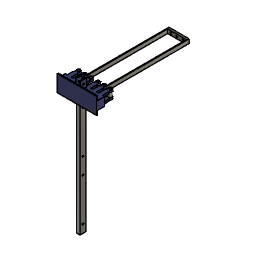
Modelo Dinamica De Estructuras (Autodesk Fusion 360 design; units mm, degrees)
Autodesk Fusion 360 part; units mm, degrees
note: some values were not read from the file. Set by a fixed rule: which sketch regions a step uses.
sketch "Boceto1" plane through (0, 0, 0) normal (0, 0, 1) x (1, 0, 0)
  circle A0 centre (0, 0) radius 2.65
  circle A1 centre (48, 0) radius 2.65
  circle A2 centre (0, 0) radius 5
  circle A3 centre (48, 0) radius 5
  line L0 (-25, -8) -> (73, -8)
  line L1 (73, -8) -> (73, -18)
  line L2 (73, -18) -> (-25, -18)
  line L3 (-25, -18) -> (-25, -8)
  line L4 (0, 0) -> (-5, -8)
  line L5 (0, 0) -> (5, -8)
  line L6 (48, 0) -> (43, -8)
  line L7 (48, 0) -> (53, -8)
  line L8 (0, 0) -> (48, 0) construction
  circle A4 centre (15, 0) radius 2.65
  circle A5 centre (15, 0) radius 5
  circle A6 centre (33, 0) radius 2.65
  circle A7 centre (33, 0) radius 5
  circle A8 centre (63, 0) radius 2.65
  circle A9 centre (63, 0) radius 5
  circle A10 centre (-15, 0) radius 5
  circle A11 centre (-15, 0) radius 2.65
  line L9 (-15, 5) -> (63, 5) construction
  line L10 (-15, 2.65) -> (63, 2.65) construction
  line L11 (-15, 0) -> (0, 0) construction
  line L12 (63, 0) -> (48, 0) construction
  line L13 (-15, 0) -> (-20, -8)
  line L14 (-15, 0) -> (-10, -8)
  line L15 (15, 0) -> (10, -8)
  line L16 (15, 0) -> (20, -8)
  line L17 (33, 0) -> (28, -8)
  line L18 (33, 0) -> (38, -8)
  line L19 (63, 0) -> (58, -8)
  line L20 (63, 0) -> (68, -8)
  dimension "d1" = 5.3
  dimension "d6" = 10
  dimension "d8" = 8
  dimension "d11" = 48
  dimension "d16" = 15
  dimension "d17" = 15
  dimension "d18" = 15
  dimension "d19" = 15
  dimension "d20" = 98
  dimension "d21" = 10
  dimension "d22" = 25
  constraint coincident A0.centre A2.centre
  constraint concentric A0 A2
  constraint concentric A1 A3
  constraint horizontal L0
  constraint vertical L1
  constraint horizontal L2
  constraint vertical L3
  constraint coincident L0 L4.end
  constraint coincident L0 L5.end
  constraint coincident A1.centre A3.centre
  constraint coincident L0 L6.end
  constraint coincident L0 L7.end
  constraint parallel L5 L7
  constraint equal L4 L5
  constraint equal L6 L7
  constraint horizontal L8
  constraint coincident L8 A4.centre
  constraint concentric A4 A5
  constraint coincident L8 A6.centre
  constraint concentric A6 A7
  constraint concentric A8 A9
  constraint concentric A10 A11
  constraint coincident A10 L9.start
  constraint horizontal L9
  constraint coincident A11 L10.start
  constraint horizontal L10
  constraint tangent A0 L10
  constraint tangent A2 L9
  constraint tangent A5 L9
  constraint tangent A4 L10
  constraint tangent A6 L10
  constraint tangent A7 L9
  constraint tangent A3 L9
  constraint tangent A1 L10
  constraint tangent A8 L10
  constraint tangent A9 L9
  constraint tangent A10 L9
  constraint tangent A11 L10
  constraint coincident A10.centre A11.centre
  constraint coincident A8.centre A9.centre
  constraint horizontal L12
  constraint horizontal L11
  constraint coincident A8 L10.end
  constraint coincident A9 L9.end
  constraint coincident L0 L13.end
  constraint coincident L0 L14.end
  constraint coincident A4.centre A5.centre
  constraint coincident L0 L15.end
  constraint coincident L0 L16.end
  constraint parallel L14 L16
  constraint coincident A6.centre A7.centre
  constraint coincident L0 L17.end
  constraint parallel L15 L17
  constraint coincident L0 L18.end
  constraint parallel L16 L18
  constraint coincident L0 L19.end
  constraint parallel L17 L19
  constraint coincident L0 L20.end
  constraint parallel L18 L20
  constraint equal L13 L14
  constraint equal L4 L14
  constraint equal L15 L16
  measures "d1" diameter of A0
  measures "d6" diameter of A2
  measures "d8" distance of A0.centre L0
  measures "d11" distance of A1.centre A0.centre
  measures "d16" distance of A0.centre A10.centre
  measures "d17" distance of A0.centre A4.centre
  measures "d18" distance of A1.centre A6.centre
  measures "d19" distance of A1.centre A8.centre
  measures "d20" distance of L1.end L2.end
  measures "d21" distance of L0.start L2.end
  measures "d22" distance of A0.centre L3
extrude "Extruir1" add sketch "Boceto1" along normal blind 21 contours A0 A2 L4 L5 | A0 A2 L4 L5 | A2 L0 L4 L5 | L0 L1 L2 L3 | L0 A10 L13 L14 | L0 A5 L15 L16 | A10 A11 L13 L14 | A10 A11 L13 L14 | A4 A5 L15 L16 | A4 A5 L15 L16 | L0 A7 L17 L18 | A6 A7 L17 L18 | A6 A7 L17 L18 | A3 L0 L6 L7 | A1 A3 L6 L7 | A1 A3 L6 L7 | L0 A9 L19 L20 | A8 A9 L19 L20 | A8 A9 L19 L20 makes body 1
sketch "Boceto2" plane through (-25, 0, 0) normal (-1, 0, 0) x (0, -1, 0)
  line L0 (8, 0) -> (18, 0)
  line L1 (18, 0) -> (18, 21)
  line L2 (18, 21) -> (8, 21)
  line L3 (8, 21) -> (8, 0)
  line L4 (8, 10.5) -> (-7.6781, 10.5)
  line L5 (-7.6781, 10.5) -> (-7.6781, 5)
  line L6 (-7.6781, 5) -> (8, 5)
  line L7 (8, 5) -> (8, 10.5)
  line L8 (8, 10.5) -> (-7.9551, 10.5)
  line L9 (-7.9551, 10.5) -> (-7.9551, 16)
  line L10 (-7.9551, 16) -> (8, 16)
  line L11 (8, 16) -> (8, 10.5)
  dimension "d23" = 11
  constraint horizontal L4
  constraint vertical L5
  constraint horizontal L6
  constraint vertical L7
  constraint midpoint L3 L4.start
  constraint horizontal L8
  constraint vertical L9
  constraint horizontal L10
  constraint vertical L11
  constraint equal L7 L11
  measures "d23" distance of L6 L10
extrude "Extruir2" cut sketch "Boceto2" against normal through all contours L3 L4 L5 L6 L7 L8 | L3 L4 L8 L9 L10 L11 bodies 1
extrude "Extruir3" add sketch "Boceto1" along normal blind 1 contours A3 L0 L6 L7 bodies 1
sketch "Boceto4" plane through (0, 0, 0) normal (0, 0, -1) x (1, 0, 0)
  circle A0 centre (48, 0) radius 3
  circle A1 centre (0, 0) radius 3
  circle A2 centre (63, 0) radius 3
  circle A3 centre (15, 0) radius 3
  circle A4 centre (33, 0) radius 3
  arc A5 (-17.65, 4.24) -> (-12.35, 4.24) centre (-15, 0) ccw
  line L0 (-12.35, 4.24) -> (-10, 8)
  line L1 (-10, 8) -> (-5, 8)
  line L2 (-5, 8) -> (-2.65, 4.24)
  arc A6 (-2.65, 4.24) -> (2.65, 4.24) centre (0, 0) ccw
  line L3 (2.65, 4.24) -> (5, 8)
  line L4 (5, 8) -> (10, 8)
  line L5 (10, 8) -> (12.35, 4.24)
  arc A7 (12.35, 4.24) -> (17.65, 4.24) centre (15, 0) ccw
  line L6 (17.65, 4.24) -> (20, 8)
  line L7 (20, 8) -> (28, 8)
  line L8 (28, 8) -> (30.35, 4.24)
  arc A8 (30.35, 4.24) -> (35.65, 4.24) centre (33, 0) ccw
  line L9 (35.65, 4.24) -> (38, 8)
  line L10 (38, 8) -> (43, 8)
  line L11 (43, 8) -> (45.35, 4.24)
  arc A9 (45.35, 4.24) -> (50.65, 4.24) centre (48, 0) ccw
  line L12 (50.65, 4.24) -> (53, 8)
  line L13 (53, 8) -> (58, 8)
  line L14 (58, 8) -> (60.35, 4.24)
  arc A10 (60.35, 4.24) -> (65.65, 4.24) centre (63, 0) ccw
  line L15 (65.65, 4.24) -> (68, 8)
  line L16 (68, 8) -> (73, 8)
  line L17 (73, 8) -> (73, 18)
  line L18 (73, 18) -> (-25, 18)
  line L19 (-25, 18) -> (-25, 8)
  line L20 (-25, 8) -> (-20, 8)
  line L21 (-20, 8) -> (-17.65, 4.24)
  circle A11 centre (-15, 0) radius 3
  circle A12 centre (48, 13) radius 4
  circle A13 centre (0, 13) radius 4
  line L22 (48, 0) -> (48, 13) construction
  line L23 (0, 0) -> (0, 13) construction
  line L24 (48, 13) -> (0, 13) construction
  dimension "d36" = 5.2
  dimension "d37" = 8
  dimension "d38" = 8
  constraint coincident A0.centre A9.centre
  constraint coincident A12.centre L22.end
  constraint coincident A1.centre A6.centre
  constraint coincident A13.centre L23.end
  constraint vertical L23
  constraint vertical L22
  constraint horizontal L24
  measures "d37" diameter of A12
  measures "d38" diameter of A13
extrude "Extruir5" [suppressed]
sketch "Boceto5" plane through (0, 0, 0) normal (0, 0, -1) x (1, 0, 0)
  circle A0 centre (48, 0) radius 2.65
  circle A1 centre (0, 0) radius 2.65
  circle A2 centre (63, 0) radius 2.65
  circle A3 centre (15, 0) radius 2.65
  circle A4 centre (33, 0) radius 2.65
  arc A5 (-17.65, 4.24) -> (-12.35, 4.24) centre (-15, 0) ccw
  line L0 (-12.35, 4.24) -> (-10, 8)
  line L1 (-10, 8) -> (-5, 8)
  line L2 (-5, 8) -> (-2.65, 4.24)
  arc A6 (-2.65, 4.24) -> (2.65, 4.24) centre (0, 0) ccw
  line L3 (2.65, 4.24) -> (5, 8)
  line L4 (5, 8) -> (10, 8)
  line L5 (10, 8) -> (12.35, 4.24)
  arc A7 (12.35, 4.24) -> (17.65, 4.24) centre (15, 0) ccw
  line L6 (17.65, 4.24) -> (20, 8)
  line L7 (20, 8) -> (28, 8)
  line L8 (28, 8) -> (30.35, 4.24)
  arc A8 (30.35, 4.24) -> (35.65, 4.24) centre (33, 0) ccw
  line L9 (35.65, 4.24) -> (38, 8)
  line L10 (38, 8) -> (43, 8)
  line L11 (43, 8) -> (45.35, 4.24)
  arc A9 (45.35, 4.24) -> (50.65, 4.24) centre (48, 0) ccw
  line L12 (50.65, 4.24) -> (53, 8)
  line L13 (53, 8) -> (58, 8)
  line L14 (58, 8) -> (60.35, 4.24)
  arc A10 (60.35, 4.24) -> (65.65, 4.24) centre (63, 0) ccw
  line L15 (65.65, 4.24) -> (68, 8)
  line L16 (68, 8) -> (73, 8)
  line L17 (73, 8) -> (73, 18)
  line L18 (73, 18) -> (-25, 18)
  line L19 (-25, 18) -> (-25, 8)
  line L20 (-25, 8) -> (-20, 8)
  line L21 (-20, 8) -> (-17.65, 4.24)
  circle A11 centre (-15, 0) radius 2.65
  line L22 (73, 18) -> (-25, 18)
  line L23 (-25, 18) -> (-25, 8)
  line L24 (-25, 8) -> (73, 8)
  line L25 (73, 8) -> (73, 18)
  constraint horizontal L22
  constraint vertical L23
  constraint horizontal L24
  constraint vertical L25
  constraint coincident L19.end L20.start
  constraint coincident L17.end L18.start
extrude "Extruir6" add sketch "Boceto5" along normal blind 50 separate body contours L1 L4 L7 L10 L13 L16 L17 L18 L19 L20 L22 L23 L24 L25 makes body 2
pattern_linear "Patrón R2" count 3 spacing 80 along (0, 0, -1) of bodies 1 makes body 3 at (40.3333, -18, -73) makes body 4 at (40.3333, -18, -153)
pattern_linear "Patrón R3" count 2 spacing 80 along (0, 0, -1) of bodies 2 makes body 5
sketch "Boceto6" plane through (0, 0, -160) normal (0, 0, -1) x (1, 0, 0)
  circle A0 centre (48, 13) radius 4
  circle A1 centre (0, 13) radius 4
  circle A2 centre (48, 0) radius 3
  circle A3 centre (0, 0) radius 3
  circle A4 centre (63, 0) radius 3
  circle A5 centre (15, 0) radius 3
  circle A6 centre (33, 0) radius 3
  arc A7 (-17.65, 4.24) -> (-12.35, 4.24) centre (-15, 0) ccw
  line L0 (-12.35, 4.24) -> (-10, 8)
  line L1 (-10, 8) -> (-5, 8)
  line L2 (-5, 8) -> (-2.65, 4.24)
  arc A8 (-2.65, 4.24) -> (2.65, 4.24) centre (0, 0) ccw
  line L3 (2.65, 4.24) -> (5, 8)
  line L4 (5, 8) -> (10, 8)
  line L5 (10, 8) -> (12.35, 4.24)
  arc A9 (12.35, 4.24) -> (17.65, 4.24) centre (15, 0) ccw
  line L6 (17.65, 4.24) -> (20, 8)
  line L7 (20, 8) -> (28, 8)
  line L8 (28, 8) -> (30.35, 4.24)
  arc A10 (30.35, 4.24) -> (35.65, 4.24) centre (33, 0) ccw
  line L9 (35.65, 4.24) -> (38, 8)
  line L10 (38, 8) -> (43, 8)
  line L11 (43, 8) -> (45.35, 4.24)
  arc A11 (45.35, 4.24) -> (50.65, 4.24) centre (48, 0) ccw
  line L12 (50.65, 4.24) -> (53, 8)
  line L13 (53, 8) -> (58, 8)
  line L14 (58, 8) -> (60.35, 4.24)
  arc A12 (60.35, 4.24) -> (65.65, 4.24) centre (63, 0) ccw
  line L15 (65.65, 4.24) -> (68, 8)
  line L16 (68, 8) -> (73, 8)
  line L17 (73, 8) -> (73, 18)
  line L18 (73, 18) -> (-25, 18)
  line L19 (-25, 18) -> (-25, 8)
  line L20 (-25, 8) -> (-20, 8)
  line L21 (-20, 8) -> (-17.65, 4.24)
  circle A13 centre (-15, 0) radius 3
  circle A14 centre (63, 0) radius 3
  circle A15 centre (48, 0) radius 3
  circle A16 centre (33, 0) radius 3
  circle A17 centre (15, 0) radius 3
  circle A18 centre (0, 0) radius 3
  circle A19 centre (-15, 0) radius 3
  circle A20 centre (0, 13) radius 4
  circle A21 centre (48, 13) radius 4
extrude "Extruir7" [suppressed]
sketch "Boceto7" plane through (0, 0, 16) normal (0, 0, -1) x (1, 0, 0)
  arc A0 (60.35, 4.24) -> (65.65, 4.24) centre (63, 0) ccw
  circle A1 centre (63, 0) radius 2.65
  circle A2 centre (48, 0) radius 2.65
  arc A3 (45.35, 4.24) -> (50.65, 4.24) centre (48, 0) ccw
  arc A4 (30.35, 4.24) -> (35.65, 4.24) centre (33, 0) ccw
  circle A5 centre (33, 0) radius 2.65
  arc A6 (12.35, 4.24) -> (17.65, 4.24) centre (15, 0) ccw
  circle A7 centre (15, 0) radius 2.65
  arc A8 (-2.65, 4.24) -> (2.65, 4.24) centre (0, 0) ccw
  circle A9 centre (0, 0) radius 2.65
  arc A10 (-17.65, 4.24) -> (-12.35, 4.24) centre (-15, 0) ccw
  circle A11 centre (-15, 0) radius 2.65
  arc A12 (60.456, 4.0704) -> (60.4559, 4.0703) centre (63, 0) ccw
  arc A13 (60.4559, 4.0703) -> (60.456, 4.0704) centre (57.912, 8.1408) ccw
  circle A14 centre (48, 0) radius 4.8
  circle A15 centre (33, 0) radius 4.8
  circle A16 centre (15, 0) radius 4.8
  circle A17 centre (0, 0) radius 4.8
  circle A18 centre (-15, 0) radius 4.8
  line L0 (63, 0) -> (-15, 0) construction
  line L1 (58.4404, -1.5) -> (52.5596, -1.5)
  line L2 (58.4404, 1.5) -> (52.5596, 1.5)
  line L3 (43.4404, -1.5) -> (37.5596, -1.5)
  line L4 (43.4404, 1.5) -> (37.5596, 1.5)
  line L5 (10.4404, -1.5) -> (4.5596, -1.5)
  line L6 (10.4404, 1.5) -> (4.5596, 1.5)
  line L7 (-4.5596, -1.5) -> (-10.4404, -1.5)
  line L8 (-4.5596, 1.5) -> (-10.4404, 1.5)
  line L9 (48, -4.8) -> (0, -4.8) construction
  line L10 (0, -4.8) -> (0, -204.8) construction
  line L11 (0, -204.8) -> (48, -204.8)
  line L12 (48, -204.8) -> (48, -4.8) construction
  line L13 (47, -204.8) -> (47, -4.6947)
  line L14 (49, -204.8) -> (49, -4.6947)
  line L15 (1, -204.8) -> (1, -4.6947)
  line L16 (-1, -204.8) -> (-1, -4.6947)
  line L17 (49, -204.8) -> (-1, -204.8)
  line L18 (-1, -204.8) -> (-1, -210)
  line L19 (-1, -210) -> (49, -210)
  line L20 (49, -210) -> (49, -204.8)
  line L21 (65.65, 4.24) -> (68, 8)
  line L22 (68, 8) -> (58, 8)
  line L23 (58, 8) -> (60.35, 4.24)
  line L24 (35.65, 4.24) -> (38, 8)
  line L25 (38, 8) -> (28, 8)
  line L26 (28, 8) -> (30.35, 4.24)
  line L27 (17.65, 4.24) -> (20, 8)
  line L28 (20, 8) -> (10, 8)
  line L29 (10, 8) -> (12.35, 4.24)
  line L30 (-12.35, 4.24) -> (-10, 8)
  line L31 (-10, 8) -> (-20, 8)
  line L32 (-20, 8) -> (-17.65, 4.24)
  line L33 (50.65, 4.24) -> (53, 8)
  line L34 (53, 8) -> (43, 8)
  line L35 (43, 8) -> (45.35, 4.24)
  line L36 (2.65, 4.24) -> (5, 8)
  line L37 (5, 8) -> (-5, 8)
  line L38 (-5, 8) -> (-2.65, 4.24)
  circle A19 centre (63, 0) radius 4.8
  dimension "d56" = 3
  dimension "d58" = 200
  dimension "d59" = 2
  dimension "d60" = 1
  dimension "d61" = 2
  dimension "d62" = 1
  dimension "d63" = 5.2
  constraint concentric A2 A14
  constraint equal A12 A14
  constraint equal A14 A15
  constraint equal A15 A16
  constraint equal A16 A17
  constraint equal A17 A18
  constraint coincident A0.centre A1.centre
  constraint coincident A10.centre A11.centre
  constraint coincident A12 L1.start
  constraint coincident A14 L1.end
  constraint horizontal L1
  constraint coincident A12 L2.start
  constraint coincident A14 L2.end
  constraint parallel L1 L2
  constraint coincident A14 L3.start
  constraint coincident A15 L3.end
  constraint parallel L2 L3
  constraint coincident A14 L4.start
  constraint coincident A15 L4.end
  constraint horizontal L4
  constraint coincident A16 L5.start
  constraint coincident A17 L5.end
  constraint horizontal L5
  constraint coincident A16 L6.start
  constraint coincident A17 L6.end
  constraint parallel L5 L6
  constraint coincident A17 L7.start
  constraint coincident A18 L7.end
  constraint parallel L6 L7
  constraint coincident A17 L8.start
  constraint coincident A18 L8.end
  constraint parallel L7 L8
  constraint symmetric L0 L1 L2
  constraint symmetric L0 L3 L4
  constraint symmetric L0 L5 L6
  constraint symmetric L0 L7 L8
  constraint collinear L1 L3
  constraint collinear L3 L5
  constraint collinear L5 L7
  constraint horizontal L9
  constraint vertical L10
  constraint horizontal L11
  constraint vertical L12
  constraint coincident A14 L9.start
  constraint coincident A2.centre L12
  constraint coincident A8.centre L10
  constraint perpendicular L11 L13
  constraint parallel L12 L14
  constraint vertical L15
  constraint parallel L10 L16
  constraint coincident A14 L13.end
  constraint coincident A14 L14.end
  constraint coincident A17 L15.end
  constraint coincident A17 L16.end
  constraint coincident L11 L15.start
  constraint coincident L11 L13.start
  constraint horizontal L17
  constraint vertical L18
  constraint horizontal L19
  constraint vertical L20
  constraint collinear L11 L17
  constraint concentric A0 A12
  constraint tangent A12 A13
  constraint concentric A12 A19
  constraint equal A15 A19
  measures "d56" distance of L1 L2
  measures "d58" distance of L9.start L11.end
  measures "d59" distance of L13 L14
  measures "d60" distance of L12 L13
  measures "d61" distance of L15 L16
  measures "d62" distance of L10 L15
  measures "d63" distance of L14.start L19.end
extrude "Extruir8" add sketch "Boceto7" along normal blind 10 separate body contours A0 A12 L1 L2 A19 | A0 A3 L1 L2 | A12 A19 | A3 A14 L1 L2 | A14 | A3 L11 L13 L14 L17 | A3 A14 L13 L14 | A3 A14 L3 L4 | L11 L17 L18 L19 L20 | A3 A4 L3 L4 | A4 A15 L3 L4 | A8 L11 L15 L16 L17 | A15 | A8 A17 L15 L16 | A8 A17 L5 L6 | A6 A8 L5 L6 | A17 | A8 A10 L7 L8 | A8 A17 L7 L8 | A6 A16 L5 L6 | A10 A18 L7 L8 | A16 | A18 makes body 6
sketch "Boceto8" plane through (0, 210, 0) normal (0, 1, 0) x (-1, 0, 0)
  line L0 (1, 16) -> (-49, 16)
  line L1 (-49, 16) -> (-49, 6)
  line L2 (-49, 6) -> (1, 6)
  line L3 (1, 6) -> (1, 16)
  line L4 (-49, 11) -> (1, 11) construction
  circle A0 centre (-39, 11) radius 2.6
  circle A1 centre (-9, 11) radius 2.6
  dimension "d66" = 5.2
  dimension "d67" = 5.2
  dimension "d68" = 10
  dimension "d69" = 30
  constraint midpoint L1 L4.start
  constraint midpoint L3 L4.end
  constraint coincident L4 A0.centre
  constraint coincident L4 A1.centre
  measures "d66" diameter of A0
  measures "d67" diameter of A1
  measures "d68" distance of L1 A0.centre
  measures "d69" distance of A0.centre A1.centre
extrude "Extruir9" [suppressed]
extrude "Extruir10" add sketch "Boceto7" along normal blind 20 separate body contours A14 | A3 L11 L13 L14 L17 | A3 A14 L13 L14 | L11 L17 L18 L19 L20 | A8 L11 L15 L16 L17 | A8 A17 L15 L16 | A17 makes body 7
sketch "Boceto9" plane through (0, 59.8, 0) normal (0, 1, 0) x (-1, 0, 0)
  line L0 (1, 25.5) -> (-49, 25.5)
  line L1 (-49, 25.5) -> (-49, 5.5)
  line L2 (-49, 5.5) -> (1, 5.5)
  line L3 (1, 5.5) -> (1, 25.5)
  line L4 (-49, 15.5) -> (1, 15.5) construction
  circle A0 centre (-39, 15.5) radius 2.5
  circle A1 centre (-9, 15.5) radius 2.5
  dimension "d75" = 5.2
  dimension "d76" = 5.2
  dimension "d77" = 10
  dimension "d78" = 30
  constraint midpoint L1 L4.start
  constraint midpoint L3 L4.end
  constraint coincident L4 A0.centre
  constraint coincident L4 A1.centre
  measures "d77" distance of L1 A0.centre
  measures "d78" distance of A0.centre A1.centre
extrude "Extruir11" [suppressed]
pattern_linear "Patrón R4" count 3 spacing 80 along (0, 0, -1) of bodies 7 makes body 8 at (-1, 138.1663, -70.6667) makes body 9 at (-1, 138.1663, -150.6667)
sketch "Boceto10" plane through (49, 0, 0) normal (1, 0, 0) x (0, 1, 0)
  line L0 (59.8, 25.5) -> (4.6947, 25.5)
  line L1 (4.6947, 25.5) -> (4.6947, 5.5)
  line L2 (4.6947, 5.5) -> (59.8, 5.5)
  line L3 (59.8, 5.5) -> (59.8, 25.5)
  line L4 (59.8, 25.5) -> (55.2846, 25.5)
  line L5 (55.2846, 25.5) -> (55.2846, 5.5)
  line L6 (55.2846, 5.5) -> (59.8, 5.5)
  line L7 (59.8, 5.5) -> (59.8, 25.5)
  constraint horizontal L4
  constraint vertical L5
  constraint horizontal L6
  constraint vertical L7
  constraint coincident L2 L5.end
  constraint coincident L0.start L3.end
extrude "Extruir12" [suppressed]
hole "Agujero1" [suppressed]
sketch "Boceto11" plane through (49, 0, 0) normal (1, 0, 0) x (0, 1, 0)
  line L0 (210, 16) -> (4.6947, 16)
  line L1 (4.6947, 16) -> (4.6947, 6)
  line L2 (4.6947, 6) -> (210, 6)
  line L3 (210, 6) -> (210, 16)
  line L4 (55, 75) -> (60, 75)
  line L5 (210, 16) -> (204.8, 16)
  line L6 (204.8, 16) -> (204.8, -4)
  line L7 (204.8, -4) -> (210, -4)
  line L8 (210, -4) -> (210, 16)
  dimension "d100" = 5.2
  constraint horizontal L4
  constraint horizontal L5
  constraint vertical L6
  constraint horizontal L7
  constraint vertical L8
  constraint coincident L0.start L3.end
  measures "d100" distance of L0.start L5.end
extrude "Extruir13" [suppressed]
sketch "Boceto13" plane through (0, 210, 0) normal (0, 1, 0) x (-1, 0, 0)
  line L0 (1, 16) -> (-59, 16)
  line L1 (-59, 16) -> (-59, 6)
  line L2 (-59, 6) -> (1, 6)
  line L3 (1, 6) -> (1, 16)
  line L4 (-59, 16) -> (-59, 11)
  line L5 (-59, 11) -> (1, 11)
  line L6 (-49, 6) -> (-49, 16)
  line L7 (-49, 16) -> (-49, 6)
  point P0 (-55.75, 11)
  dimension "d122" = 6.75
  constraint coincident L0.end L1.start
  constraint midpoint L1 L4.end
  constraint midpoint L3 L5.end
  constraint coincident L5 P0
  measures "d122" distance of P0 L7
hole "Agujero2" [suppressed]
sketch "Boceto12" plane through (0, -18, 0) normal (0, -1, 0) x (1, 0, 0)
  line L0 (-25, 0) -> (73, 0)
  line L1 (73, 0) -> (73, 21)
  line L2 (73, 21) -> (-25, 21)
  line L3 (-25, 21) -> (-25, 0)
  line L4 (-25, 21) -> (-24, 21)
  line L5 (-24, 21) -> (-24, -9)
  line L6 (-24, -9) -> (-25, -9)
  line L7 (-25, -9) -> (-25, 21)
  dimension "d106" = 1
  constraint horizontal L4
  constraint vertical L5
  constraint horizontal L6
  constraint vertical L7
  constraint coincident L2.end L3.start
  measures "d106" distance of L2.end L4.end
extrude "Extruir14" [suppressed]
moveface "MoveFace1" [suppressed]
extrude "Extruir15" [suppressed]
extrude "Extruir16" [suppressed]
extrude "Extruir17" [suppressed]
extrude "Extruir18" add 1 faces at (40.3333, -18, 7) along direction (0, -1, 0) blind 25 on bodies 1 bodies 1
extrude "Extruir19" cut 1 faces at (61.3333, -8, 12.3333) along direction (0, -1, 0) blind 15 on bodies 1 bodies 1
sketch "Boceto14" plane through (0, 210, 0) normal (0, 1, 0) x (-1, 0, 0)
  line L0 (1, 16) -> (-49, 16)
  line L1 (-49, 16) -> (-49, 6)
  line L2 (-49, 6) -> (1, 6)
  line L3 (1, 6) -> (1, 16)
  line L4 (1, 6) -> (-49, 16)
  circle A0 centre (-24, 11) radius 2.15
  circle A1 centre (-39, 11) radius 2.15
  circle A2 centre (-9, 11) radius 2.15
  dimension "d123" = 4.3
  dimension "d126" = 15
  dimension "d127" = 0
  constraint coincident L2.end L3.start
  constraint coincident L0.end L1.start
  constraint midpoint L4 A0.centre
  measures "d123" diameter of A0
extrude "Extruir20" cut sketch "Boceto14" against normal blind 10 contours L4 A0 | L4 A0 | A1 | A2 bodies 6
sketch "Boceto15" plane through (49, 0, 0) normal (1, 0, 0) x (0, 1, 0)
  line L0 (210, 16) -> (4.6947, 16)
  line L1 (4.6947, 16) -> (4.6947, 6)
  line L2 (4.6947, 6) -> (210, 6)
  line L3 (210, 6) -> (210, 16)
  line L4 (204.8, 16) -> (4.6947, 16)
  line L5 (4.6947, 16) -> (4.6947, 6)
  line L6 (4.6947, 6) -> (204.8, 6)
  line L7 (204.8, 6) -> (204.8, 16)
  line L8 (204.8, 11) -> (4.6947, 11) construction
  line L9 (204.8, 6.005) -> (4.6947, 6.005)
  line L10 (4.6947, 6.005) -> (4.6947, 15.995)
  line L11 (4.6947, 15.995) -> (204.8, 15.995)
  line L12 (204.8, 15.995) -> (204.8, 6.005)
  line L13 (204.8, 6.005) -> (4.6947, 15.995) construction
  line L14 (4.6947, 6.005) -> (204.8, 15.995) construction
  point P0 (104.7473, 11)
  dimension "d130" = 9.99
  constraint midpoint L7 L8.start
  constraint midpoint L5 L8.end
  constraint horizontal L9
  constraint perpendicular L9 L10
  constraint parallel L9 L11
  constraint parallel L10 L12
  constraint coincident L13 P0
  constraint coincident L14 P0
  constraint coincident L7 L9.start
  constraint midpoint L8 P0
  measures "d130" distance of L9 L11
extrude "Extruir21" cut sketch "Boceto15" against normal blind 75 contours L0 L1 L4 L5 L7 L11 | L1 L2 L5 L6 L7 L9 bodies 6
sketch "Boceto16" plane through (0, 0, 21) normal (0, 0, 1) x (-1, 0, 0)
  line L0 (20, 23) -> (25, 23)
  line L1 (25, 23) -> (25, 43)
  line L2 (25, 43) -> (-73, 43)
  line L3 (-73, 43) -> (-73, 23)
  line L4 (-73, 23) -> (-68, 23)
  line L5 (-68, 23) -> (-68, 8)
  line L6 (-68, 8) -> (-65.65, 4.24)
  arc A0 (-65.65, 4.24) -> (-60.35, 4.24) centre (-63, 0) ccw
  line L7 (-60.35, 4.24) -> (-58, 8)
  line L8 (-58, 8) -> (-58, 23)
  line L9 (-58, 23) -> (-53, 23)
  line L10 (-53, 23) -> (-53, 8)
  line L11 (-53, 8) -> (-50.65, 4.24)
  arc A1 (-50.65, 4.24) -> (-45.35, 4.24) centre (-48, 0) ccw
  line L12 (-45.35, 4.24) -> (-43, 8)
  line L13 (-43, 8) -> (-43, 23)
  line L14 (-43, 23) -> (-38, 23)
  line L15 (-38, 23) -> (-38, 8)
  line L16 (-38, 8) -> (-35.65, 4.24)
  arc A2 (-35.65, 4.24) -> (-30.35, 4.24) centre (-33, 0) ccw
  line L17 (-30.35, 4.24) -> (-28, 8)
  line L18 (-28, 8) -> (-28, 23)
  line L19 (-28, 23) -> (-20, 23)
  line L20 (-20, 23) -> (-20, 8)
  line L21 (-20, 8) -> (-17.65, 4.24)
  arc A3 (-17.65, 4.24) -> (-12.35, 4.24) centre (-15, 0) ccw
  line L22 (-12.35, 4.24) -> (-10, 8)
  line L23 (-10, 8) -> (-10, 23)
  line L24 (-10, 23) -> (-5, 23)
  line L25 (-5, 23) -> (-5, 8)
  line L26 (-5, 8) -> (-2.65, 4.24)
  arc A4 (-2.65, 4.24) -> (2.65, 4.24) centre (0, 0) ccw
  line L27 (2.65, 4.24) -> (5, 8)
  line L28 (5, 8) -> (5, 23)
  line L29 (5, 23) -> (10, 23)
  line L30 (10, 23) -> (10, 8)
  line L31 (10, 8) -> (12.35, 4.24)
  arc A5 (12.35, 4.24) -> (17.65, 4.24) centre (15, 0) ccw
  line L32 (17.65, 4.24) -> (20, 8)
  line L33 (20, 8) -> (20, 23)
  circle A6 centre (-15, 0) radius 2.65
  circle A7 centre (-63, 0) radius 2.65
  circle A8 centre (15, 0) radius 2.65
  circle A9 centre (-48, 0) radius 2.65
  circle A10 centre (0, 0) radius 2.65
  circle A11 centre (-33, 0) radius 2.65
  line L34 (25, 23) -> (-73, 43)
  line L35 (-73, 23) -> (25, 43)
  line L36 (-19, 40.5) -> (-29, 40.5)
  line L37 (-29, 40.5) -> (-29, 25.5)
  line L38 (-29, 25.5) -> (-19, 25.5)
  line L39 (-19, 25.5) -> (-19, 40.5)
  line L40 (-19, 40.5) -> (-29, 25.5) construction
  line L41 (-29, 40.5) -> (-19, 25.5) construction
  line L42 (-30.5, 25.5) -> (-17.5, 25.5)
  line L43 (-17.5, 25.5) -> (-17.5, 40.5)
  line L44 (-17.5, 40.5) -> (-30.5, 40.5)
  line L45 (-30.5, 40.5) -> (-30.5, 25.5)
  line L46 (-30.5, 25.5) -> (-17.5, 40.5) construction
  line L47 (-17.5, 25.5) -> (-30.5, 40.5) construction
  point P0 (-24, 33)
  point P1 (-24, 33)
  dimension "d134" = 10
  dimension "d135" = 15
  dimension "d136" = 13
  dimension "d137" = 15
  constraint coincident L0.end L1.start
  constraint coincident L2.end L3.start
  constraint coincident L3.end L4.start
  constraint coincident L1.end L2.start
  constraint horizontal L36
  constraint perpendicular L36 L37
  constraint parallel L36 L38
  constraint parallel L37 L39
  constraint coincident L40 P1
  constraint coincident L41 P1
  constraint midpoint L35 P1
  constraint horizontal L42
  constraint perpendicular L42 L43
  constraint parallel L42 L44
  constraint parallel L43 L45
  constraint coincident L46 P1
  constraint coincident L47 P1
  constraint coincident P1 P0
  measures "d134" distance of L37.end L38.end
  measures "d135" distance of L36.end L37.end
  measures "d136" distance of L43.end L44.end
  measures "d137" distance of L42.end L43.end
extrude "Extruir22" add sketch "Boceto16" along normal blind 20 contours L34 L39 L42 L43 | L34 L35 L39 L43 | L35 L39 L43 L44 | L34 L37 L44 L45 | L34 L35 L37 L45 | L35 L37 L42 L45 bodies 1
sketch "Boceto17" plane through (0, 0, 21) normal (0, 0, 1) x (-1, 0, 0)
extrude "Extruir23" cut sketch "Boceto16" against normal blind 30 contours L34 L35 L37 L38 L39 L42 | L34 L35 L39 | L34 L35 L36 L37 L39 L44 | L34 L35 L37 bodies 1
sketch "Boceto18" plane through (17.5, 0, 0) normal (-1, 0, 0) x (0, -1, 0)
  line L0 (25.5, 21) -> (40.5, 21)
  line L1 (40.5, 21) -> (40.5, 41)
  line L2 (40.5, 41) -> (25.5, 41)
  line L3 (25.5, 41) -> (25.5, 21)
  line L4 (40.5, 41) -> (25.5, 21)
  circle A0 centre (33, 31) radius 2.15
  dimension "d142" = 4.3
  constraint coincident L1.end L2.start
  constraint coincident L0.start L3.end
  constraint midpoint L4 A0.centre
  measures "d142" diameter of A0
extrude "Extruir24" cut sketch "Boceto18" against normal blind 30 contours L4 A0 | L4 A0 bodies 1
sketch "Boceto19" plane through (0, 0, 0) normal (0, 0, -1) x (1, 0, 0)
  circle A0 centre (48, 0) radius 2.65
  line L0 (-25, 23) -> (-20, 23)
  line L1 (-20, 23) -> (-20, 8)
  line L2 (-20, 8) -> (-17.65, 4.24)
  arc A1 (-17.65, 4.24) -> (-12.35, 4.24) centre (-15, 0) ccw
  line L3 (-12.35, 4.24) -> (-10, 8)
  line L4 (-10, 8) -> (-10, 23)
  line L5 (-10, 23) -> (-5, 23)
  line L6 (-5, 23) -> (-5, 8)
  line L7 (-5, 8) -> (-2.65, 4.24)
  arc A2 (-2.65, 4.24) -> (2.65, 4.24) centre (0, 0) ccw
  line L8 (2.65, 4.24) -> (5, 8)
  line L9 (5, 8) -> (5, 23)
  line L10 (5, 23) -> (10, 23)
  line L11 (10, 23) -> (10, 8)
  line L12 (10, 8) -> (12.35, 4.24)
  arc A3 (12.35, 4.24) -> (17.65, 4.24) centre (15, 0) ccw
  line L13 (17.65, 4.24) -> (20, 8)
  line L14 (20, 8) -> (20, 23)
  line L15 (20, 23) -> (28, 23)
  line L16 (28, 23) -> (28, 8)
  line L17 (28, 8) -> (30.35, 4.24)
  arc A4 (30.35, 4.24) -> (35.65, 4.24) centre (33, 0) ccw
  line L18 (35.65, 4.24) -> (38, 8)
  line L19 (38, 8) -> (38, 23)
  line L20 (38, 23) -> (43, 23)
  line L21 (43, 23) -> (43, 8)
  line L22 (43, 8) -> (45.35, 4.24)
  arc A5 (45.35, 4.24) -> (50.65, 4.24) centre (48, 0) ccw
  line L23 (50.65, 4.24) -> (53, 8)
  line L24 (53, 8) -> (53, 23)
  line L25 (53, 23) -> (58, 23)
  line L26 (58, 23) -> (58, 8)
  line L27 (58, 8) -> (60.35, 4.24)
  arc A6 (60.35, 4.24) -> (65.65, 4.24) centre (63, 0) ccw
  line L28 (65.65, 4.24) -> (68, 8)
  line L29 (68, 8) -> (68, 23)
  line L30 (68, 23) -> (73, 23)
  line L31 (73, 23) -> (73, 43)
  line L32 (73, 43) -> (-25, 43)
  line L33 (-25, 43) -> (-25, 23)
  circle A7 centre (15, 0) radius 2.65
  circle A8 centre (63, 0) radius 2.65
  circle A9 centre (-15, 0) radius 2.65
  circle A10 centre (0, 0) radius 2.65
  circle A11 centre (33, 0) radius 2.65
  line L34 (29, 40.5) -> (29, 25.5)
  line L35 (29, 25.5) -> (19, 25.5)
  line L36 (19, 25.5) -> (19, 40.5)
  line L37 (19, 40.5) -> (29, 40.5)
  line L38 (19.254, 40.0837) -> (28.754, 40.0837)
  line L39 (28.754, 40.0837) -> (28.754, 25.5837)
  line L40 (28.754, 25.5837) -> (19.254, 25.5837)
  line L41 (19.254, 25.5837) -> (19.254, 40.0837)
  line L42 (19, 40.5) -> (29, 40.5)
  line L43 (29, 40.5) -> (29, 25.5)
  line L44 (29, 25.5) -> (19, 25.5)
  line L45 (19, 25.5) -> (19, 40.5)
  dimension "d152" = 14.5
  dimension "d153" = 9.5
  measures "d152" distance of L38 L40
  measures "d153" distance of L39 L41
extrude "Extruir25" add sketch "Boceto19" along normal blind 290 separate body contours L38 L39 L40 L41 makes body 10
sketch "Boceto20" plane through (19.254, 0, 0) normal (-1, 0, 0) x (0, -1, 0)
  line L0 (40.0837, 0) -> (25.5837, 0)
  line L1 (25.5837, 0) -> (25.5837, -290)
  line L2 (25.5837, -290) -> (40.0837, -290)
  line L3 (40.0837, -290) -> (40.0837, 0)
  line L4 (25.5837, -290) -> (40.0837, 0)
  line L5 (34.9837, -257.5) -> (34.9837, -32.5)
  arc A0 (34.9837, -32.5) -> (30.6837, -32.5) centre (32.8337, -32.5) ccw
  line L6 (30.6837, -32.5) -> (30.6837, -257.5)
  arc A1 (30.6837, -257.5) -> (34.9837, -257.5) centre (32.8337, -257.5) ccw
  line L7 (32.8337, -257.5) -> (32.8337, -32.5) construction
  point P0 (32.8337, -145)
  dimension "d148" = 4.3
  dimension "d149" = 225
  constraint coincident L1.end L2.start
  constraint coincident L0.start L3.end
  constraint tangent L5 A0
  constraint tangent A0 L6
  constraint parallel L5 L6
  constraint tangent L6 A1
  constraint tangent L5 A1
  constraint perpendicular L0 L7
  constraint midpoint L4 P0
  constraint midpoint L7 P0
  measures "d148" diameter of A0
  measures "d149" distance of A1.centre A0.centre
extrude "Extruir26" [suppressed]
sketch "Boceto21" plane through (28.754, 0, 0) normal (1, 0, 0) x (0, 1, 0)
  line L0 (-25.5837, 0) -> (-40.0837, 0)
  line L1 (-40.0837, 0) -> (-40.0837, -290)
  line L2 (-40.0837, -290) -> (-25.5837, -290)
  line L3 (-25.5837, -290) -> (-25.5837, 0)
  line L4 (-25.5837, 0) -> (-40.0837, 0)
  line L5 (-40.0837, 0) -> (-40.0837, -290)
  line L6 (-40.0837, -290) -> (16.4012, -290)
  line L7 (16.4012, -290) -> (-25.5837, 0)
  line L8 (-25.5837, 0) -> (-40.0837, -290)
  line L9 (-40.0837, 0) -> (-25.5837, -290)
  circle A0 centre (-32.8337, -145) radius 2.175
  circle A1 centre (-32.8337, -270) radius 2.175
  circle A2 centre (-32.8337, -20) radius 2.175
  dimension "d154" = 4.35
  dimension "d157" = 0
  dimension "d158" = 125
  constraint horizontal L4
  constraint horizontal L6
  constraint coincident L1.end L2.start
  constraint coincident L0.start L3.end
  constraint coincident L0.end L1.start
  constraint coincident L2.end L3.start
  constraint midpoint L9 A0.centre
  measures "d154" diameter of A0
extrude "Extruir27" cut sketch "Boceto21" against normal blind 9.5 contours A1 | A2 bodies 10
sketch "Boceto22" plane through (0, 0, 21) normal (0, 0, 1) x (-1, 0, 0)
  circle A0 centre (-33, 0) radius 2.65
  circle A1 centre (0, 0) radius 2.65
  circle A2 centre (-48, 0) radius 2.65
  circle A3 centre (15, 0) radius 2.65
  circle A4 centre (-63, 0) radius 2.65
  circle A5 centre (-15, 0) radius 2.65
  line L0 (20, 23) -> (25, 23)
  line L1 (25, 23) -> (25, 43)
  line L2 (25, 43) -> (-73, 43)
  line L3 (-73, 43) -> (-73, 23)
  line L4 (-73, 23) -> (-68, 23)
  line L5 (-68, 23) -> (-68, 8)
  line L6 (-68, 8) -> (-65.65, 4.24)
  arc A6 (-65.65, 4.24) -> (-60.35, 4.24) centre (-63, 0) ccw
  line L7 (-60.35, 4.24) -> (-58, 8)
  line L8 (-58, 8) -> (-58, 23)
  line L9 (-58, 23) -> (-53, 23)
  line L10 (-53, 23) -> (-53, 8)
  line L11 (-53, 8) -> (-50.65, 4.24)
  arc A7 (-50.65, 4.24) -> (-45.35, 4.24) centre (-48, 0) ccw
  line L12 (-45.35, 4.24) -> (-43, 8)
  line L13 (-43, 8) -> (-43, 23)
  line L14 (-43, 23) -> (-38, 23)
  line L15 (-38, 23) -> (-38, 8)
  line L16 (-38, 8) -> (-35.65, 4.24)
  arc A8 (-35.65, 4.24) -> (-30.35, 4.24) centre (-33, 0) ccw
  line L17 (-30.35, 4.24) -> (-28, 8)
  line L18 (-28, 8) -> (-28, 23)
  line L19 (-28, 23) -> (-20, 23)
  line L20 (-20, 23) -> (-20, 8)
  line L21 (-20, 8) -> (-17.65, 4.24)
  arc A9 (-17.65, 4.24) -> (-12.35, 4.24) centre (-15, 0) ccw
  line L22 (-12.35, 4.24) -> (-10, 8)
  line L23 (-10, 8) -> (-10, 23)
  line L24 (-10, 23) -> (-5, 23)
  line L25 (-5, 23) -> (-5, 8)
  line L26 (-5, 8) -> (-2.65, 4.24)
  arc A10 (-2.65, 4.24) -> (2.65, 4.24) centre (0, 0) ccw
  line L27 (2.65, 4.24) -> (5, 8)
  line L28 (5, 8) -> (5, 23)
  line L29 (5, 23) -> (10, 23)
  line L30 (10, 23) -> (10, 8)
  line L31 (10, 8) -> (12.35, 4.24)
  arc A11 (12.35, 4.24) -> (17.65, 4.24) centre (15, 0) ccw
  line L32 (17.65, 4.24) -> (20, 8)
  line L33 (20, 8) -> (20, 23)
  line L34 (-19, 25.5) -> (-29, 25.5)
  line L35 (-29, 25.5) -> (-30.5, 25.5)
  line L36 (-30.5, 25.5) -> (-30.5, 40.5)
  line L37 (-30.5, 40.5) -> (-29, 40.5)
  line L38 (-29, 40.5) -> (-19, 40.5)
  line L39 (-19, 40.5) -> (-17.5, 40.5)
  line L40 (-17.5, 40.5) -> (-17.5, 25.5)
  line L41 (-17.5, 25.5) -> (-19, 25.5)
  line L42 (25, 43) -> (-73, 43)
  line L43 (-73, 43) -> (-73, 40.5)
  line L44 (-73, 40.5) -> (25, 40.5)
  line L45 (25, 40.5) -> (25, 43)
  constraint horizontal L42
  constraint vertical L43
  constraint horizontal L44
  constraint vertical L45
  constraint coincident L3 L43.end
  constraint coincident L1.end L2.start
extrude "Extruir28" add sketch "Boceto22" along normal blind 10 contours L1 L2 L3 L37 L38 L39 L42 L43 L44 L45 bodies 1
sketch "Boceto23" plane through (0, 0, 0) normal (0, 0, -1) x (1, 0, 0)
  line L0 (19, 40.5) -> (29, 40.5)
  line L1 (29, 40.5) -> (29, 25.5)
  line L2 (29, 25.5) -> (19, 25.5)
  line L3 (19, 25.5) -> (19, 40.5)
  circle A0 centre (48, 0) radius 2.65
  line L4 (-25, 23) -> (-20, 23)
  line L5 (-20, 23) -> (-20, 8)
  line L6 (-20, 8) -> (-17.65, 4.24)
  arc A1 (-17.65, 4.24) -> (-12.35, 4.24) centre (-15, 0) ccw
  line L7 (-12.35, 4.24) -> (-10, 8)
  line L8 (-10, 8) -> (-10, 23)
  line L9 (-10, 23) -> (-5, 23)
  line L10 (-5, 23) -> (-5, 8)
  line L11 (-5, 8) -> (-2.65, 4.24)
  arc A2 (-2.65, 4.24) -> (2.65, 4.24) centre (0, 0) ccw
  line L12 (2.65, 4.24) -> (5, 8)
  line L13 (5, 8) -> (5, 23)
  line L14 (5, 23) -> (10, 23)
  line L15 (10, 23) -> (10, 8)
  line L16 (10, 8) -> (12.35, 4.24)
  arc A3 (12.35, 4.24) -> (17.65, 4.24) centre (15, 0) ccw
  line L17 (17.65, 4.24) -> (20, 8)
  line L18 (20, 8) -> (20, 23)
  line L19 (20, 23) -> (28, 23)
  line L20 (28, 23) -> (28, 8)
  line L21 (28, 8) -> (30.35, 4.24)
  arc A4 (30.35, 4.24) -> (35.65, 4.24) centre (33, 0) ccw
  line L22 (35.65, 4.24) -> (38, 8)
  line L23 (38, 8) -> (38, 23)
  line L24 (38, 23) -> (43, 23)
  line L25 (43, 23) -> (43, 8)
  line L26 (43, 8) -> (45.35, 4.24)
  arc A5 (45.35, 4.24) -> (50.65, 4.24) centre (48, 0) ccw
  line L27 (50.65, 4.24) -> (53, 8)
  line L28 (53, 8) -> (53, 23)
  line L29 (53, 23) -> (58, 23)
  line L30 (58, 23) -> (58, 8)
  line L31 (58, 8) -> (60.35, 4.24)
  arc A6 (60.35, 4.24) -> (65.65, 4.24) centre (63, 0) ccw
  line L32 (65.65, 4.24) -> (68, 8)
  line L33 (68, 8) -> (68, 23)
  line L34 (68, 23) -> (73, 23)
  line L35 (73, 23) -> (73, 43)
  line L36 (73, 43) -> (-25, 43)
  line L37 (-25, 43) -> (-25, 23)
  circle A7 centre (15, 0) radius 2.65
  circle A8 centre (63, 0) radius 2.65
  circle A9 centre (-15, 0) radius 2.65
  circle A10 centre (0, 0) radius 2.65
  circle A11 centre (33, 0) radius 2.65
  line L38 (73, 43) -> (-25, 43)
  line L39 (-25, 43) -> (-25, 40.5)
  line L40 (-25, 40.5) -> (73, 40.5)
  line L41 (73, 40.5) -> (73, 43)
  constraint horizontal L38
  constraint vertical L39
  constraint horizontal L40
  constraint vertical L41
  constraint coincident L37 L39.end
  constraint coincident L35.end L36.start
extrude "Extruir29" add sketch "Boceto23" along normal blind 10 contours L0 L35 L36 L37 L38 L39 L40 L41 bodies 1
chamfer "Chaflán1" [suppressed]
sketch "Boceto24" plane through (28.754, 0, 0) normal (1, 0, 0) x (0, 1, 0)
  circle A0 centre (-32.8337, -270) radius 2.175
  line L0 (-25.5837, 0) -> (-40.0837, 0)
  line L1 (-40.0837, 0) -> (-40.0837, -290)
  line L2 (-40.0837, -290) -> (-25.5837, -290)
  line L3 (-25.5837, -290) -> (-25.5837, 0)
  line L4 (-25.5837, 0) -> (-40.0837, 0)
  line L5 (-40.0837, 0) -> (-40.0837, -290)
  line L6 (-40.0837, -290) -> (-25.5837, -290)
  line L7 (-25.5837, -290) -> (-25.5837, 0)
  line L8 (-25.5837, 0) -> (-40.0837, -290)
  line L9 (-25.5837, -290) -> (-40.0837, 0)
  circle A1 centre (-32.8337, -145) radius 2.175
  circle A2 centre (-32.8337, -165) radius 2.175
  circle A3 centre (-32.8337, -125) radius 2.175
  circle A4 centre (-32.8337, -20) radius 2.175
  dimension "d169" = 4.35
  dimension "d180" = 0
  dimension "d181" = 20
  constraint horizontal L4
  constraint horizontal L6
  constraint vertical L7
  constraint coincident L1.end L2.start
  constraint coincident L0.start L3.end
  constraint coincident L2.end L3.start
  constraint coincident L0.end L1.start
  constraint midpoint L8 A1.centre
  measures "d169" diameter of A1
extrude "Extruir30" cut sketch "Boceto24" against normal blind 9.5 contours L8 A3 | L8 L9 A3 | L9 A3 | L8 L9 A2 | L9 A2 | L8 A2 bodies 10
hidden bodies 2 3 4 5 7 8 9
equation "d2 = Ancho_Marco_Plano + 11 mm"
equation "d23 = Ancho_Marco_Plano + 1 mm"
equation "d38 = d37"
equation "d58 = Altura_Marco_Plano"
equation "d64 = Ancho_Marco_Plano"
equation "d67 = d66"
equation "Altura_Marco_Plano = 200 mm"
equation "Ancho_Marco_Plano = 10 mm"
equation "d122 = ( 13.5 / 2 ) * 1 mm"
equation "d130 = Ancho_Columna"
equation "Ancho_Columna = 9.99 mm"
equation "d140 = -3 * Ancho_Marco_Plano"
equation "d146 = Largo_Pasador"
equation "d152 = Alto_Pasador"
equation "d153 = Ancho_Pasador"
equation "d154 = Diametro_Pasador"
equation "d159 = -Ancho_Pasador"
equation "Ancho_Pasador = 9.5 mm"
equation "Alto_Pasador = 14.5 mm"
equation "Largo_Pasador = 290 mm"
equation "d169 = Diametro_Pasador"
equation "d182 = -Ancho_Pasador"
equation "Diametro_Pasador = 4.35 mm"
named bodies: "Base Marco Plano", "Marco Plano", "Pasador"
